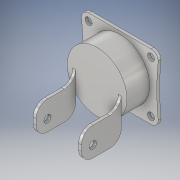
# Autodesk Inventor part: CastorBase
Saved by Autodesk Inventor 2018 (Build 220112000, 112)
## iProperties
Created: 2018-01-12
Part Number: CastorBase
Material: Stainless Steel
Document SubType Name: Modeling
Designer: Kyle
Density: 8 g/cm^3
Appearance: Aluminum - Polished
Author: Kyle
Autodesk Inventor part; units mm, degrees
ref_plane "YZ Plane" through (0, 0, 0) normal (1, 0, 0) x (0, 1, 0)
ref_plane "XZ Plane" through (0, 0, 0) normal (0, 1, 0) x (-1, 0, 0)
ref_plane "XY Plane" through (0, 0, 0) normal (0, 0, 1) x (1, 0, 0)
sketch "Sketch1" plane through (0, 0, 0) normal (0, 0, 1) x (1, 0, 0)
  arc A0 (0, 3.175) -> (-3.175, 0) centre (0, 0) ccw
  arc A1 (-3.175, -22.86) -> (0, -26.035) centre (0, -22.86) ccw
  line L0 (0, -26.035) -> (27.94, -26.035)
  line L1 (0, 3.175) -> (27.94, 3.175)
  circle A2 centre (0, -22.86) radius 1.5875
  circle A3 centre (27.94, -22.86) radius 1.5875
  circle A4 centre (0, 0) radius 1.5875
  circle A5 centre (27.94, 0) radius 1.5875
  arc A6 (-3.175, -22.86) -> (-3.175, 0) centre (-101.9139, -11.43) ccw
  arc A7 (31.115, 0) -> (31.115, -22.86) centre (133.6675, -11.43) ccw
  arc A8 (27.94, -26.035) -> (31.115, -22.86) centre (27.94, -22.86) ccw
  arc A9 (31.115, 0) -> (27.94, 3.175) centre (27.94, 0) ccw
  point P0 (30.48, -11.43)
  point P1 (-2.54, -11.43)
  point P2 (-3.0961, -0.7033)
  dimension "d0" = 27.94
  dimension "d1" = 22.86
  dimension "d3" = 6.35
  dimension "d4" = 6.35
  dimension "d6" = 33.02
  dimension "d7" = 11.43
  dimension "d8" = 2.54
  dimension "d9" = 3.175
  dimension "d10" = 3.175
  dimension "d11" = 3.175
  dimension "d12" = 3.175
  dimension "d34" = 27.94
  dimension "d35" = 22.86
  dimension "d36" = 0
  dimension "d37" = 0
  constraints: 14 point on circle, 10 centre point, 9 coincident, 4 end point, 2 tangent, 1 horizontal, 1 parallel
  measures "d0" distance of point (0, 0) point (27.94, 0)
  measures "d1" distance of point (27.94, -22.86) point (27.94, 0)
  measures "d3" diameter of A0
  measures "d4" diameter of A1
  measures "d6" distance of point (30.48, -11.43) point (-2.54, -11.43)
  measures "d7" vertical distance of point (0, 0) point (-2.54, -11.43)
  measures "d8" horizontal distance of point (-2.54, -11.43) point (0, 0)
  measures "d9" diameter of A5
  measures "d10" diameter of A4
  measures "d11" diameter of A2
  measures "d12" diameter of A3
  measures "d34" distance of A1.centre A8.centre
  measures "d35" distance of A1.centre point (0, 0)
  measures "d36" horizontal distance of A1.centre point (0, 0)
  measures "d37" vertical distance of point (-2.54, -11.43) point (30.48, -11.43)
extrude "Extrusion1" add sketch "Sketch1" along normal blind 1.27
sketch "Sketch2" plane through (0, 0, 1.27) normal (0, 0, 1) x (1, 0, 0)
  circle A0 centre (13.97, -11.43) radius 13.335
  point P0 (0, 0)
  dimension "d15" = 26.67
  dimension "d16" = 13.97
  dimension "d17" = 11.43
  constraints: 1 centre point
  measures "d15" diameter of A0
  measures "d16" horizontal distance of point (0, 0) A0.centre
  measures "d17" vertical distance of point (0, 0) A0.centre
extrude "Extrusion2" add sketch "Sketch2" along normal blind 10.16
sketch "Sketch3" plane through (13.97, -11.43, 11.43) normal (0, 0, 1) x (1, 0, 0)
  line L0 (9.525, -5.08) -> (10.795, -5.08)
  line L1 (10.795, -5.08) -> (10.795, -17.78)
  line L2 (10.795, -17.78) -> (9.525, -17.78)
  line L3 (9.525, -17.78) -> (9.525, -5.08)
  line L4 (-10.795, -5.08) -> (-9.525, -5.08)
  line L5 (-9.525, -5.08) -> (-9.525, -17.78)
  line L6 (-9.525, -17.78) -> (-10.795, -17.78)
  line L7 (-10.795, -17.78) -> (-10.795, -5.08)
  circle A0 centre (0, 0) radius 13.335 projected
  point P0 (-13.97, 11.43)
  point P1 (-13.335, 0)
  dimension "d20" = 19.05
  dimension "d21" = 1.27
  dimension "d22" = 1.27
  dimension "d23" = 3.81
  dimension "d24" = 5.08
  dimension "d25" = 12.7
  constraints: 16 end point, 4 parallel, 2 collinear, 2 horizontal, 2 perpendicular, 1 horizontal alignment, 2 other
  measures "d20" distance between parallel lines of L5 L3
  measures "d21" distance of L0.start L0.end
  measures "d22" distance of L4.start L4.end
  measures "d23" distance from line of point (-13.335, 0) L5
  measures "d24" distance from line of point (0, 0) L0
  measures "d25" distance of L0.end L1.end
extrude "Extrusion3" add sketch "Sketch3" along normal blind 17.78 contours L0 L1 A0 L3 | A0 L1 L2 L3 | A0 L7 L4 L5 | L5 L6 L7 A0
sketch "Sketch4" plane through (24.765, -29.21, 11.43) normal (1, 0, 0) x (0, 0, -1)
  line L0 (0, 0) -> (-17.78, 0) projected
  line L1 (-17.78, 0) -> (-17.78, 12.7) projected
  circle A0 centre (-12.7, 5.08) radius 1.5875
  point P0 (11.43, 29.21)
  dimension "d28" = 5.08
  dimension "d29" = 5.08
  dimension "d30" = 3.175
  constraints: 1 centre point, 1 coincident
  measures "d28" distance from line of L0 point (-12.7, 5.08)
  measures "d29" distance from line of L1 point (-12.7, 5.08)
  measures "d30" diameter of A0
extrude "Extrusion4" cut sketch "Sketch4" against normal blind 50.8
fillet "Fillet1" radius 5.08 8 edges at (24.13, -29.21, 29.21) (3.81, -29.21, 29.21) (24.13, -16.51, 29.21) (3.81, -16.51, 29.21) (3.81, -16.51, 11.43) (24.13, -16.51, 11.43) (3.81, -29.21, 11.43) (24.13, -29.21, 11.43)
body "Solid1"
